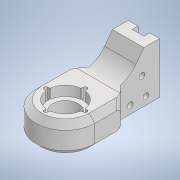
# Autodesk Inventor part: dog_bone_1
Saved by Autodesk Inventor 2020 (Build 240168000, 168)
## iProperties
Created: 2019-05-15
Part Number: dog_bone_1
Material: Generic
Document SubType Name: Modeling
Designer: psrob
Density: 1 g/cm^3
Appearance: Default
Author: psrob
Autodesk Inventor part; units mm, degrees
ref_plane "YZ Plane" through (0, 0, 0) normal (1, 0, 0) x (0, 1, 0)
ref_plane "XZ Plane" through (0, 0, 0) normal (0, 1, 0) x (-1, 0, 0)
ref_plane "XY Plane" through (0, 0, 0) normal (0, 0, 1) x (1, 0, 0)
sketch "Sketch1" plane through (0, 0, 0) normal (0, 1, 0) x (-1, 0, 0)
  circle A0 centre (0, 0) radius 15
  circle A1 centre (0, 0) radius 5
  line L0 (15, 0) -> (-15, 0)
  line L1 (-15, 0) -> (-15, -40)
  line L2 (-15, -40) -> (15, -40)
  line L3 (15, -40) -> (15, 0)
  dimension "d1" = 30
  dimension "d0" = 10
  dimension "d2" = 30
  dimension "d3" = 40
  constraints: 8 end point, 2 coincident, 2 parallel, 1 centre point, 1 horizontal, 1 perpendicular, 3 other
  measures "d0" diameter of A1
  measures "d2" distance of L1.end L2.end
  measures "d3" distance of L2.end L0.start
extrude "Extrusion1" add sketch "Sketch1" along normal blind 10 contours L0 A1 A0 | L3 L2 L1 A0 | A0 L0 A1
sketch "Sketch2" plane through (15, 0, -40) normal (0, 0, -1) x (-1, 0, 0)
  line L0 (0, 0) -> (30, 0) projected
  line L1 (30, 0) -> (30, 10) projected
  line L2 (0, 10) -> (30, 10) projected
  line L3 (0, 0) -> (0, 10) projected
  line L4 (30, 0) -> (0, 0)
  line L5 (0, 0) -> (0, 40)
  line L6 (0, 40) -> (30, 40)
  line L7 (30, 40) -> (30, 0)
  point P0 (15, 0)
  dimension "d6" = 30
  dimension "d7" = 40
  constraints: 8 end point, 2 parallel, 1 horizontal, 1 perpendicular
  measures "d6" distance of L5.end L6.end
  measures "d7" distance of L4.end L5.end
extrude "Extrusion2" add sketch "Sketch2" along normal blind 10
thicken "Thicken1" operation add thickness 5 both sides no extend neighbours yes toward (0, 0, 1) faces at (-5, 26.6667, -50)
sketch "Sketch3" plane through (0, 0, 0) normal (0, -1, 0) x (1, 0, 0)
  line L0 (15, 0) -> (15, -45) projected
  arc A0 (15, 0) -> (-15, 0) centre (0, 0) ccw projected
  line L1 (-15, -45) -> (-15, 0) projected
  line L2 (15, -45) -> (-15, -45) projected
  circle A1 centre (0, 0) radius 5 projected
  line L3 (-15, -45) -> (15, -45) projected
  line L4 (-15, -45) -> (-8, -45)
  line L5 (-8, -45) -> (-8, -20)
  line L6 (15, -40) -> (15, -45) projected
  line L7 (15, -45) -> (8, -45)
  line L8 (8, -45) -> (8, -20)
  line L9 (-8, -20) -> (-15, -20)
  line L10 (-15, -20) -> (-15, -13)
  line L11 (-15, -13) -> (-8, -13)
  line L12 (-8, -13) -> (-8, -20)
  line L13 (8, -20) -> (15, -20)
  line L14 (15, -20) -> (15, -13)
  line L15 (15, -13) -> (8, -13)
  line L16 (8, -13) -> (8, -20)
  line L17 (-15, -13) -> (-8, -20)
  line L18 (8, -20) -> (15, -13)
  dimension "d12" = 7
  dimension "d13" = 25
  dimension "d14" = 7
  dimension "d15" = 25
  dimension "d16" = 7
  dimension "d17" = 7
  dimension "d18" = 7
  dimension "d19" = 7
  constraints: 28 end point, 4 parallel, 4 perpendicular, 2 horizontal, 2 point on line
  measures "d12" distance of L1.start L4.end
  measures "d13" distance of L4.end L5.end
  measures "d14" distance of L0.end L7.end
  measures "d15" distance of L7.end L8.end
  measures "d16" distance of L10.end L11.end
  measures "d17" distance of L9.end L10.end
  measures "d18" distance of L15.end L14.end
  measures "d19" distance of L14.end L13.end
extrude "Extrusion3" cut sketch "Sketch3" against normal blind 50 contours L0 L13 L18 | L0 L2 L8 L13 | L17 L9 L1 | L9 L5 L2 L1
thicken "Thicken2" operation add thickness 5 both sides no extend neighbours yes toward (0, 0, 1) faces at (-2.6667, 20, -40)
thicken "Thicken3" operation add thickness 5 both sides no extend neighbours yes toward (0, 0, 1) faces at (-2.6667, 26.6667, -45)
sketch "Sketch4" plane through (-8, 0, -20) normal (-1, 0, 0) x (0, 0, 1)
  line L0 (-20, 40) -> (-15, 40) projected
  line L1 (-20, 0) -> (-20, 40) projected
  line L2 (0, 0) -> (-20, 0) projected
  line L3 (0, 0) -> (0, 10) projected
  line L4 (-15, 10) -> (0, 10) projected
  line L5 (-15, 40) -> (-15, 10) projected
  line L6 (-15, 40) -> (-15, 30)
  line L7 (-15, 10) -> (-15, 40) projected
  line L8 (-15, 30) -> (0, 10)
  point P0 (20, 0)
  dimension "d26" = 10
  constraints: 4 end point, 1 point on line
  measures "d26" distance of L0.end L6.end
extrude "Extrusion4" add sketch "Sketch4" against normal up to surface (16 mm away) contours L8 L4 L5
sketch "Sketch5" plane through (-8, 0, -40) normal (-1, 0, 0) x (0, 0, 1)
  line L0 (0, 40) -> (5, 40) projected
  line L1 (0, 0) -> (0, 40) projected
  line L2 (20, 0) -> (0, 0) projected
  line L3 (20, 0) -> (20, 10) projected
  line L4 (20, 10) -> (5, 30) projected
  line L5 (5, 40) -> (5, 30) projected
  line L6 (20, 0) -> (0, 0) projected
  line L7 (0, 0) -> (0, 20)
  line L8 (0, 40) -> (0, 0) projected
  line L9 (0, 20) -> (20, 0)
  point P0 (40, 0)
  dimension "d29" = 20
  constraints: 4 end point, 1 midpoint
  measures "d29" distance of L1.start L7.end
extrude "Extrusion5" cut sketch "Sketch5" against normal up to surface (16 mm away) contours L9 L2 L1
sketch "Sketch6" plane through (-8, 40, -40) normal (-1, 0, 0) x (0, 0, 1)
  line L0 (0, -20) -> (20, -40) projected
  line L1 (20, -40) -> (20, -30) projected
  line L2 (20, -30) -> (5, -10) projected
  line L3 (5, 0) -> (5, -10) projected
  line L4 (0, 0) -> (5, 0) projected
  line L5 (0, -20) -> (0, 0) projected
  line L6 (0, -20) -> (10, -20)
  line L7 (10, -20) -> (10, -30)
  line L8 (10, -30) -> (0, -30)
  line L9 (0, -30) -> (0, -20)
  point P0 (40, -40)
  dimension "d32" = 10
  dimension "d33" = 10
  constraints: 8 end point, 2 parallel, 1 horizontal, 1 perpendicular
  measures "d32" distance of L7.end L8.end
  measures "d33" distance of L6.end L7.end
extrude "Extrusion6" add sketch "Sketch6" against normal up to surface (16 mm away) contours L0 L8 L9
sketch "Sketch7" plane through (-8, 10, -40) normal (0, -1, 0) x (1, 0, 0)
  line L0 (16, 10) -> (16, 0) projected
  line L1 (0, 10) -> (16, 10) projected
  line L2 (0, 0) -> (0, 10) projected
  line L3 (0, 0) -> (16, 0) projected
  line L4 (11, -3) -> (5, -3)
  line L5 (5, -3) -> (5, 3)
  line L6 (5, 3) -> (11, 3)
  line L7 (11, 3) -> (11, -3)
  line L8 (0, 0) -> (16, 0) projected
  line L9 (11, -3) -> (5, 3) construction
  line L10 (5, -3) -> (11, 3) construction
  line L11 (0, 0) -> (16, 0) projected
  point P0 (8, 40)
  point P1 (8, 0)
  dimension "d36" = 6
  dimension "d37" = 6
  constraints: 12 end point, 3 midpoint, 2 parallel, 2 perpendicular
  measures "d36" distance of L4.start L4.end
  measures "d37" distance of L6.end L4.start
extrude "Extrusion7" cut sketch "Sketch7" against normal up to surface (30 mm away) contours L7 L4 L5 L3 | L3 L5 L6 L7
sketch "Sketch9" plane through (-8, 40, -40) normal (-1, 0, 0) x (0, 0, 1)
  line L0 (8.0217, 14.8834) -> (8.0217, 33.2834) projected
  line L1 (8.0217, 33.2834) -> (20.0216, 46.8834) projected
  line L2 (20, 46.8834) -> (20.0216, 46.8834) projected
  line L3 (20, 54.8834) -> (20, 46.8834) projected
  line L4 (0, 54.8834) -> (20, 54.8834) projected
  line L5 (0, 14.8834) -> (0, 54.8834) projected
  line L6 (8.0217, 14.8834) -> (0, 14.8834) projected
  line L7 (10, -30) -> (20, -40) projected
  line L8 (20, -40) -> (20, -30) projected
  line L9 (20, -30) -> (5, -10) projected
  line L10 (5, 0) -> (5, -10) projected
  line L11 (0, 0) -> (5, 0) projected
  line L12 (0, -30) -> (0, 0) projected
  line L13 (0, -30) -> (10, -30) projected
  line L14 (8.0217, 17.8834) -> (8.0217, -14.0289)
  line L15 (20, -30) -> (5, -10) projected
  line L16 (8.0217, -14.0289) -> (0, -14.0289)
  line L17 (0, -30) -> (0, 0) projected
  line L18 (0, -14.0289) -> (0, 0)
  line L19 (5, 0) -> (5, -10) projected
  line L20 (5, -10) -> (8.0217, -14.0289)
  ellipse E0 centre (10.0217, 50.8834) end of major axis (10.0217, 49.3834) minor radius 1.5 projected
  ellipse E1 centre (8.0149, 40.8834) end of major axis (8.0149, 39.3834) minor radius 1.5 projected
  point P0 (40, -40)
  point P1 (8.0217, -14.0289)
  constraints: 8 end point, 2 collinear, 2 point on line, 1 perpendicular, 1 vertical
extrude "Extrusion9" cut sketch "Sketch9" against normal blind 20 contours L12 L11 L10 L9 L16
sketch "Sketch10" plane through (8, 0, -20) normal (1, 0, 0) x (0, 0, -1)
  line L0 (20, 25.9711) -> (11.9783, 25.9711) projected
  line L1 (11.9783, 25.9711) -> (0, 10) projected
  line L2 (0, 0) -> (0, 10) projected
  line L3 (0, 0) -> (10, 10) projected
  line L4 (10, 10) -> (20, 10) projected
  line L5 (20, 10) -> (20, 25.9711) projected
  line L6 (0, 0) -> (20, 0)
  line L7 (20, 10) -> (20, 25.9711) projected
  line L8 (20, 0) -> (20, 10)
  point P0 (-20, 0)
  constraints: 4 end point, 1 horizontal, 1 perpendicular
extrude "Extrusion10" add sketch "Sketch10" against normal up to surface (16 mm away) contours L8 L6 L3 L4
thicken "Thicken4" operation add thickness 20 both sides no extend neighbours yes toward (0, -1, 0) faces at (1, 10, -39)
sketch "Sketch11" plane through (0, 0, 0) normal (0, -1, 0) x (1, 0, 0)
  circle A0 centre (0, 0) radius 6.5
  dimension "d49" = 13
  constraints: 1 centre point, 1 coincident
  measures "d49" diameter of A0
extrude "Extrusion11" cut sketch "Sketch11" against normal blind 20
sketch "Sketch12" plane through (0, 10, 0) normal (0, 1, 0) x (1, 0, 0)
  circle A0 centre (0, 0) radius 6.5 projected
  line L0 (8, 20) -> (-8, 20) projected
  line L1 (-8, 20) -> (-15, 13) projected
  line L2 (-15, 13) -> (-15, 0) projected
  arc A1 (-15, 0) -> (15, 0) centre (0, 0) ccw projected
  line L3 (15, 0) -> (15, 13) projected
  line L4 (15, 13) -> (8, 20) projected
  circle A2 centre (0, 0) radius 15
  circle A3 centre (0, 0) radius 9
  point P0 (15, 0)
  dimension "d52" = 30
  dimension "d53" = 18
  constraints: 2 centre point, 2 coincident
  measures "d52" diameter of A2
  measures "d53" diameter of A3
extrude "Extrusion12" add sketch "Sketch12" along normal blind 5 contours A1 A2
sketch "Sketch14" plane through (0, 15, 0) normal (0, 1, 0) x (1, 0, 0)
  line L0 (15, 13) -> (8, 20) projected
  line L1 (8, 20) -> (-8, 20) projected
  line L2 (-8, 20) -> (-15, 13) projected
  line L3 (-15, 13) -> (-15, 0) projected
  arc A0 (15, 0) -> (-15, 0) centre (0, 0) ccw projected
  line L4 (15, 0) -> (15, 13) projected
  circle A1 centre (0, 0) radius 15 projected
  circle A2 centre (0, 0) radius 9 projected
  line L5 (-8, 20) -> (8, 20)
  line L6 (8, 20) -> (8, 28)
  line L7 (8, 28) -> (-8, 28)
  line L8 (-8, 28) -> (-8, 20)
  dimension "d67" = 16
  dimension "d68" = 8
  constraints: 8 end point, 2 parallel, 1 horizontal, 1 perpendicular
  measures "d67" distance of L7.end L6.end
  measures "d68" distance of L6.end L5.end
extrude "Extrusion14" add sketch "Sketch14" against normal up to surface (5 mm away) contours L4 A0 L3 L2 L1 L0 | L1 L8 L7 L6
fillet "Fillet5" radius 14 1 edges at (0, 15, -23.75)
chamfer "Chamfer2" distance 3 angle 45 6 edges at (0, 0, 15) (15, 0, -6.5) (-15, 0, -6.5) (-15, 15, -6.5) (0, 15, 15) (15, 15, -6.5)
fillet "Fillet6" radius 3 4 edges at (-13.5, 13.5, -14.5) (-13.5, 1.5, -14.5) (13.5, 13.5, -14.5) (13.5, 1.5, -14.5)
sketch "Sketch15" plane through (8, 0, -20) normal (1, 0, 0) x (0, 0, -1)
  line L0 (0, 15.3825) -> (0, 0) projected
  line L1 (0, 0) -> (20, 0) projected
  line L2 (20, 0) -> (20, 25.9711) projected
  line L3 (20, 25.9711) -> (11.9783, 25.9711) projected
  line L4 (11.9783, 25.9711) -> (7.95, 20.6) projected
  arc A0 (0, 15.3825) -> (7.95, 20.6) centre (-3.25, 29) ccw projected
  line L5 (17, 0) -> (17, 25.9711) projected
  line L6 (20, 0) -> (20, 4)
  line L7 (20, 0) -> (20, 25.9711) projected
  line L8 (20, 4) -> (13, 4)
  line L9 (13, 4) -> (5, 4)
  circle A1 centre (5, 4) radius 1.5
  circle A2 centre (13, 4) radius 1.5
  point P0 (-20, 0)
  dimension "d76" = 4
  dimension "d77" = 7
  dimension "d78" = 8
  dimension "d79" = 3
  dimension "d80" = 3
  constraints: 6 end point, 2 centre point, 2 coincident, 2 point on line, 1 perpendicular
  measures "d76" distance of L1.end L6.end
  measures "d77" distance of L6.end L8.end
  measures "d78" distance of L8.end L9.end
  measures "d79" diameter of A1
  measures "d80" diameter of A2
extrude "Extrusion15" cut sketch "Sketch15" against normal blind 20 contours A2 L9 L8 | L8 L9 A2 | A1
sketch "Sketch17" plane through (8, 0, -20) normal (1, 0, 0) x (0, 0, -1)
  circle A0 centre (13, 4) radius 1.5 projected
  circle A1 centre (5, 4) radius 1.5 projected
  line L0 (0, 15.3825) -> (0, 0) projected
  line L1 (0, 0) -> (20, 0) projected
  line L2 (20, 0) -> (20, 25.9711) projected
  line L3 (20, 25.9711) -> (11.9783, 25.9711) projected
  line L4 (11.9783, 25.9711) -> (7.95, 20.6) projected
  arc A2 (0, 15.3825) -> (7.95, 20.6) centre (-3.25, 29) ccw projected
  line L5 (13, 4) -> (13, 14)
  line L6 (17, 0) -> (17, 25.9711) projected
  line L7 (13, 14) -> (11, 14)
  circle A3 centre (11, 14) radius 1.5
  point P0 (-20, 0)
  dimension "d89" = 10
  dimension "d90" = 2
  dimension "d91" = 3
  constraints: 4 end point, 1 centre point, 1 coincident, 1 horizontal, 1 vertical
  measures "d89" distance of L5.start L5.end
  measures "d90" distance of L5.end L7.end
  measures "d91" diameter of A3
extrude "Extrusion17" cut sketch "Sketch17" against normal blind 20 contours A3
sketch "Sketch18" plane through (0, 0, 0) normal (0, -1, 0) x (1, 0, 0)
  circle A0 centre (0, 0) radius 6.5 projected
  ellipse E0 centre (7.7574, -16) end of major axis (11.4316, -12.3258) minor radius 3 (9.8787, -18.1213) -> (12, -13.8787) ccw projected
  line L0 (12, 0) -> (12, -13.8787) projected
  arc A1 (12, 0) -> (-12, 0) centre (0, 0) ccw projected
  line L1 (-12, -13.8787) -> (-12, 0) projected
  ellipse E1 centre (-7.7574, -16) end of major axis (-11.4316, -12.3258) minor radius 3 (-12, -13.8787) -> (-9.8787, -18.1213) ccw projected
  line L2 (-9.8787, -18.1213) -> (-8, -20) projected
  line L3 (-8, -40) -> (-8, -20) projected
  line L4 (-3, -40) -> (-8, -40) projected
  line L5 (-3, -37) -> (-3, -40) projected
  line L6 (3, -37) -> (-3, -37) projected
  line L7 (3, -40) -> (3, -37) projected
  line L8 (8, -40) -> (3, -40) projected
  line L9 (8, -20) -> (8, -40) projected
  line L10 (8, -20) -> (9.8787, -18.1213) projected
  line L11 (0, 0) -> (10, 0)
  circle A2 centre (10, 0) radius 1
  circle A3 centre (0, 10) radius 1
  circle A4 centre (-10, 0) radius 1
  circle A5 centre (0, -10) radius 1
  dimension "d94" = 10
  dimension "d95" = 2
  dimension "d98" = 360
  constraints: 4 centre point, 2 end point, 1 coincident, 1 horizontal, 11 other
  measures "d94" distance of L11.start L11.end
  measures "d95" diameter of A2
extrude "Extrusion18" cut sketch "Sketch18" against normal blind 20 contours A2 | A3 | A4 | A5
sketch "Sketch19" plane through (0, 15, 0) normal (0, 1, 0) x (1, 0, 0)
  arc A0 (0, -9) -> (9, 0) centre (0, 0) ccw projected
  circle A1 centre (0, -10) radius 1 projected
  arc A2 (-9, 0) -> (0, -9) centre (0, 0) ccw projected
  circle A3 centre (-10, 0) radius 1 projected
  arc A4 (0, 9) -> (-9, 0) centre (0, 0) ccw projected
  circle A5 centre (0, 10) radius 1 projected
  arc A6 (9, 0) -> (0, 9) centre (0, 0) ccw projected
  circle A7 centre (10, 0) radius 1 projected
  ellipse E0 centre (7.7574, 16) end of major axis (11.4316, 12.3258) minor radius 3 (12, 13.8787) -> (10.9987, 16.75) ccw projected
  line L0 (-10.9987, 16.75) -> (10.9987, 16.75) projected
  ellipse E1 centre (-7.7574, 16) end of major axis (-11.4316, 12.3258) minor radius 3 (-10.9987, 16.75) -> (-12, 13.8787) ccw projected
  line L1 (-12, 0) -> (-12, 13.8787) projected
  arc A8 (-12, 0) -> (12, 0) centre (0, 0) ccw projected
  line L2 (12, 13.8787) -> (12, 0) projected
  circle A9 centre (10, 0) radius 1 projected
  line L3 (0, 0) -> (10, 0) construction
  line L4 (0, 1) -> (10, 1)
  line L5 (10, -1) -> (0, -1)
  arc A10 (0, 1) -> (0, -1) centre (0, 0) ccw
  arc A11 (10, -1) -> (10, 1) centre (10, 0) ccw
  line L6 (0, 0) -> (0, -10) construction
  line L7 (1, 0) -> (1, -10)
  line L8 (-1, -10) -> (-1, 0)
  arc A12 (1, 0) -> (-1, 0) centre (0, 0) ccw
  arc A13 (-1, -10) -> (1, -10) centre (0, -10) ccw
  circle A14 centre (-10, 0) radius 1 projected
  line L9 (0, 0) -> (-10, 0) construction
  line L10 (0, 1) -> (-10, 1)
  line L11 (-10, -1) -> (0, -1)
  arc A15 (0, -1) -> (0, 1) centre (0, 0) ccw
  arc A16 (-10, 1) -> (-10, -1) centre (-10, 0) ccw
  circle A17 centre (0, 10) radius 1 projected
  line L12 (0, 0) -> (0, 10) construction
  line L13 (-1, 0) -> (-1, 10)
  line L14 (1, 10) -> (1, 0)
  arc A18 (-1, 0) -> (1, 0) centre (0, 0) ccw
  arc A19 (1, 10) -> (-1, 10) centre (0, 10) ccw
  point P0 (5, 0)
  point P1 (0, -5)
  point P2 (-5, 0)
  point P3 (0, 5)
  point P4 (-1, -1)
  point P5 (1, -10)
  point P6 (1, -1)
  point P7 (1, 1)
  point P8 (-1, 1)
  constraints: 32 end point, 16 point on circle, 16 tangent, 8 centre point, 4 midpoint, 4 parallel, 3 perpendicular, 1 horizontal, 7 other
extrude "Extrusion19" cut sketch "Sketch19" against normal up to surface (5 mm away) contours A2 L8 L11 L5 L7 A0 | A0 L7 A1 | A1 | A1 L8 A2 | L5 L7 L14 L4 A6 A0 | A0 A7 L5 | L5 A15 L7 | L11 A3 A2 | A2 A4 L10 L13 L8 L11 | L8 A10 L11 | A6 L4 A7 | A7 | A10 A12 A15 | A12 L4 L14 | A3 | A3 L10 A4 | L13 L10 A10 | L10 L13 A4 A6 L14 L4 | A6 A5 L14 | L13 A5 A4 | A5
fillet "Fillet7" radius 0.5 8 edges at (8.9443, 12.5, -1) (8.9443, 12.5, 1) (1, 12.5, 8.9443) (-1, 12.5, 8.9443) (-8.9443, 12.5, 1) (-8.9443, 12.5, -1) (-1, 12.5, -8.9443) (1, 12.5, -8.9443)
sketch "Sketch20" plane through (0, 0, 0) normal (0, -1, 0) x (1, 0, 0)
  circle A0 centre (-10, 0) radius 1 projected
  circle A1 centre (0, -10) radius 1 projected
  circle A2 centre (0, 10) radius 1 projected
  circle A3 centre (10, 0) radius 1 projected
  circle A4 centre (0, 0) radius 6.5 projected
  ellipse E0 centre (7.7574, -16) end of major axis (11.4316, -12.3258) minor radius 3 (9.8787, -18.1213) -> (12, -13.8787) ccw projected
  line L0 (12, 0) -> (12, -13.8787) projected
  arc A5 (12, 0) -> (-12, 0) centre (0, 0) ccw projected
  line L1 (-12, -13.8787) -> (-12, 0) projected
  ellipse E1 centre (-7.7574, -16) end of major axis (-11.4316, -12.3258) minor radius 3 (-12, -13.8787) -> (-9.8787, -18.1213) ccw projected
  line L2 (-9.8787, -18.1213) -> (-8, -20) projected
  line L3 (-8, -40) -> (-8, -20) projected
  line L4 (-3, -40) -> (-8, -40) projected
  line L5 (-3, -37) -> (-3, -40) projected
  line L6 (3, -37) -> (-3, -37) projected
  line L7 (3, -40) -> (3, -37) projected
  line L8 (8, -40) -> (3, -40) projected
  line L9 (8, -20) -> (8, -40) projected
  line L10 (8, -20) -> (9.8787, -18.1213) projected
  line L11 (-3, -37) -> (3, -37) projected
  line L12 (0, -37) -> (0, -29)
  line L13 (0, -29) -> (0, -19)
  circle A6 centre (0, -19) radius 1.5
  circle A7 centre (0, -29) radius 1.5
  dimension "d105" = 8
  dimension "d106" = 10
  dimension "d107" = 3
  dimension "d108" = 3
  constraints: 4 end point, 2 centre point, 2 coincident, 1 midpoint, 1 point on line, 1 vertical, 2 other
  measures "d105" distance of L12.start L12.end
  measures "d106" distance of L12.end L13.end
  measures "d107" diameter of A6
  measures "d108" diameter of A7
extrude "Extrusion20" cut sketch "Sketch20" against normal blind 10 contours A7 L13 L12 | L12 L13 A7 | A6
body "Solid1"
